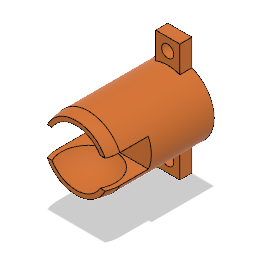
Fixateur bille (Autodesk Fusion 360 design; units mm, degrees)
Autodesk Fusion 360 part; units mm, degrees
sphere "Sphère de départ" add diameter 17 placed x (1, 0, 0) y (0, 0, -1) z (0, 1, 0) at (0, 0, 0) makes body 1
shell "Evidage sphère" thickness 1 removed faces 0 bodies 1
ref_plane "WorkPlane1" through (0, 0, 3) normal (0, 0, 1) x (1, 0, 0)
split "Section avant" by plane through (0, 0, 3) normal (0, 0, 1) bodies 1 makes body 2 at (-5.4981, 0.571, 6.4572)
delete_body "RemoveBody1" bodies 2
cylinder "Cylindre extension" add diameter 17 height -22.5 placed x (1, 0, 0) y (0, 1, 0) z (0, 0, 1) at (0, 0, 0) separate body makes body 3
sphere "Shère évidage cylindre" cut diameter 15 placed x (1, 0, 0) y (0, 0, -1) z (0, 1, 0) at (0, 0, 0) bodies 3
combine "Combine1" operation add target body 1 tool bodies 3
ref_plane "WorkPlane4" through (0, 8.5, -11.25) normal (0, 1, 0) x (1, 0, 0)
sketch "Sketch vis haut" plane through (0, 8.5, -4.25) normal (0, 1, 0) x (1, 0, 0)
  line L0 (0, 18.25) -> (0, 16.75)
  line L1 (-3, 18.25) -> (3, 18.25)
  line L2 (3, 18.25) -> (3, 15.25)
  line L3 (3, 15.25) -> (-3, 15.25)
  line L4 (-3, 15.25) -> (-3, 18.25)
  line L5 (0, 16.75) -> (0.1, 16.75)
  point P0 (0, 16.75)
  point P1 (0, 18.25)
  dimension "d72" = 1.5
  dimension "d73" = 3
  dimension "d74" = 6
  constraint coincident P1 L0.start
  constraint coincident P0 L0.end
  constraint vertical L0
  constraint horizontal L1
  constraint vertical L2
  constraint horizontal L3
  constraint vertical L4
  constraint symmetric L0 L2 L4
  constraint perpendicular L0 L5
  constraint symmetric L1 L3 L5
  measures "d72" distance of P0 L0.start
  measures "d73" distance of L1.end L2.end
  measures "d74" distance of L2 L4
extrude "Extrude vis haut" add sketch "Sketch vis haut" along normal blind 6 and the other way blind 2 separate body makes body 4
hole "Trou vis haut" at (0, 11.5, -19.5) direction (0, 0, -1) diameter 3 depth 3 tip angle 180 bodies 4
mirror "Mirroir vis" about plane through (0, 0, 0) normal (0, 1, 0) of bodies 4 makes body 5
combine "Combine2" operation add target body 1 tool bodies 4 5
sketch "Sketch13" plane through (0, 0, 3) normal (0, 0, 1) x (1, 0, 0)
  line L0 (9, 3.5) -> (-9, 3.5)
  line L1 (-9, 3.5) -> (-9, -3.5)
  line L2 (-9, -3.5) -> (9, -3.5)
  line L3 (9, -3.5) -> (9, 3.5)
  line L4 (9, 3.5) -> (-9, -3.5) construction
  line L5 (-9, 3.5) -> (9, -3.5) construction
  dimension "d54" = 7
  dimension "d55" = 18
  constraint perpendicular L0 L1
  constraint parallel L0 L2
  constraint parallel L1 L3
  constraint horizontal L0
  constraint coincident L4 origin
  constraint coincident L5 origin
  measures "d54" distance of L0.end L1.end
  measures "d55" distance of L1.end L2.end
extrude "Extrude écartement" cut sketch "Sketch13" against normal blind 10 bodies 1
named bodies: "Fixateur"
